Autodesk Inventor part; units mm, degrees
(part 3 of 3)
sketch "Skizze43" plane through (0, 0, 0) normal (0, 0, -1) x (-1, 0, 0)
  circle A0 centre (-82, 71.5) radius 1.7 projected
  circle A1 centre (-82, 71.5) radius 3
  circle A2 centre (-82, 31.5) radius 1.7 projected
  circle A3 centre (-82, 31.5) radius 3
  circle A4 centre (-82, -11.5) radius 1.7 projected
  circle A5 centre (-82, -11.5) radius 3
  circle A6 centre (-82, -51.5) radius 1.7 projected
  circle A7 centre (-82, -51.5) radius 3
  circle A8 centre (82, -51.5) radius 1.7 projected
  circle A9 centre (82, -51.5) radius 3
  circle A10 centre (82, -11.5) radius 1.7 projected
  circle A11 centre (82, -11.5) radius 3
  circle A12 centre (82, 31.5) radius 1.7 projected
  circle A13 centre (82, 31.5) radius 3
  circle A14 centre (82, 71.5) radius 1.7 projected
  circle A15 centre (82, 71.5) radius 3
  point P0 (0, 0)
  dimension "d224" = 6
  dimension "d225" = 6
  dimension "d226" = 6
  dimension "d227" = 6
  dimension "d228" = 6
  dimension "d229" = 6
  dimension "d230" = 6
  dimension "d231" = 6
  constraints: 8 centre point, 8 coincident
  measures "d224" diameter of A15
  measures "d225" diameter of A13
  measures "d226" diameter of A11
  measures "d227" diameter of A9
  measures "d228" diameter of A1
  measures "d229" diameter of A3
  measures "d230" diameter of A5
  measures "d231" diameter of A7
extrude "Extrusion27" cut sketch "Skizze43" against normal blind 10 contours A1 | A2 | A3 | A4 | A5 | A6 | A7 | A8 | A9 | A10 | A11 | A12 | A13 | A15
